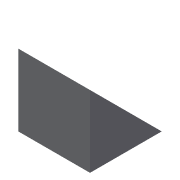
# Autodesk Inventor part: edge
Saved by Autodesk Inventor 2015 (Build 190159000, 159)
## iProperties
Created: 2016-08-26
Part Number: edge
Material: Ogólny
Document SubType Name: Modeling
Designer: EriveltonDell
Density: 1 g/cm^3
Appearance: Domyślna
Author: EriveltonDell
Autodesk Inventor part; units mm, degrees
ref_plane "YZ Plane" through (0, 0, 0) normal (1, 0, 0) x (0, 1, 0)
ref_plane "XZ Plane" through (0, 0, 0) normal (0, 1, 0) x (-1, 0, 0)
ref_plane "XY Plane" through (0, 0, 0) normal (0, 0, 1) x (1, 0, 0)
sketch "Sketch1" plane through (0, 0, 0) normal (1, 0, 0) x (0, 1, 0)
  line L0 (0, 0) -> (30, 0)
  line L1 (30, 0) -> (30, 30)
  line L2 (30, 30) -> (0, 30)
  line L3 (0, 30) -> (0, 0)
  dimension "d0" = 30
  dimension "d1" = 30
  constraints: 8 end point, 2 parallel, 1 horizontal, 1 perpendicular
  measures "d0" distance of L2.end L1.end
  measures "d1" distance of L1.end L0.end
extrude "Extrusion1" add sketch "Sketch1" along normal blind 30
chamfer "Chamfer1" distance 30 angle 45 1 edges at (15, 30, 30)
body "Solid1"
